Autodesk Fusion 360 part; units mm, degrees
(part 6 of 6)
  spline S266 degree 5 poles (46.3256, -26.1313) (46.3173, -26.12) (46.3005, -26.0976) (46.2753, -26.0639) (46.2416, -26.0191) (46.1993, -25.9633) (46.1569, -25.9077) (46.1143, -25.8522) (46.0715, -25.797) (46.0286, -25.7419) (45.9856, -25.687) (45.9424, -25.6324) (45.899, -25.5779) (45.8555, -25.5236) (45.8119, -25.4695) (45.768, -25.4156) (45.7241, -25.3619) (45.6799, -25.3084) (45.6356, -25.2552) (45.5912, -25.2021) (45.5466, -25.1492) (45.5018, -25.0966) (45.4569, -25.0441) (45.4118, -24.9919) (45.3665, -24.9399) (45.3211, -24.8881) (45.2755, -24.8365) (45.2297, -24.7851) (45.1838, -24.734) (45.1377, -24.6831) (45.0914, -24.6324) (45.045, -24.582) (44.9984, -24.5318) (44.9516, -24.4818) (44.9046, -24.4321) (44.8575, -24.3827) (44.8102, -24.3334) (44.7627, -24.2845) (44.7151, -24.2357) (44.6672, -24.1873) (44.6192, -24.1391) (44.571, -24.0912) (44.5226, -24.0435) (44.481, -24.003) (44.4491, -23.9721) (44.4268, -23.9507) (44.4144, -23.9388) (44.4117, -23.9362) knots -1 -1 -1 -1 -1 -1 -0.985714 -0.971429 -0.957143 -0.942857 -0.928571 -0.914286 -0.9 -0.885714 -0.871429 -0.857143 -0.842857 -0.828571 -0.814286 -0.8 -0.785714 -0.771429 -0.757143 -0.742857 -0.728571 -0.714286 -0.7 -0.685714 -0.671429 -0.657143 -0.642857 -0.628571 -0.614286 -0.6 -0.585714 -0.571429 -0.557143 -0.542857 -0.528571 -0.514286 -0.5 -0.485714 -0.471429 -0.457143 -0.442857 -0.428571 -0.414286 -0.4 -0.396066 -0.396066 -0.396066 -0.396066 -0.396066 -0.396066
  spline S267 degree 3 poles (44.3152, -23.3421) (44.2848, -23.3997) (44.266, -23.4627) (44.2536, -23.5923) (44.2602, -23.6577) (44.2914, -23.761) (44.309, -23.8002) (44.3538, -23.8731) (44.3808, -23.9066) (44.4117, -23.9362) knots 0 0 0 0 0.019532 0.019532 0.039064 0.039064 0.051902 0.051902 0.06474 0.06474 0.06474 0.06474
  arc A134 (44.3152, -23.3421) -> (44.5389, -22.9124) centre (0, 0) ccw
  spline S268 degree 3 poles (45.0809, -22.6507) (45.017, -22.638) (44.9513, -22.6379) (44.8235, -22.663) (44.7626, -22.6878) (44.6726, -22.7472) (44.64, -22.7753) (44.5828, -22.839) (44.5585, -22.8743) (44.5389, -22.9124) knots 0 0 0 0 0.019532 0.019532 0.039064 0.039064 0.051902 0.051902 0.06474 0.06474 0.06474 0.06474
  spline S269 degree 5 poles (45.0809, -22.6507) (45.0845, -22.6514) (45.1015, -22.6548) (45.1317, -22.6607) (45.1754, -22.6692) (45.2324, -22.68) (45.2992, -22.6923) (45.3661, -22.7043) (45.4331, -22.716) (45.5003, -22.7274) (45.5675, -22.7385) (45.6349, -22.7493) (45.7023, -22.7598) (45.7699, -22.77) (45.8375, -22.78) (45.9053, -22.7897) (45.9731, -22.799) (46.0411, -22.8081) (46.1091, -22.817) (46.1773, -22.8255) (46.2455, -22.8338) (46.3138, -22.8419) (46.3822, -22.8496) (46.4507, -22.8571) (46.5193, -22.8644) (46.5879, -22.8714) (46.6566, -22.8781) (46.7255, -22.8846) (46.7944, -22.8908) (46.8633, -22.8968) (46.9324, -22.9025) (47.0015, -22.908) (47.0707, -22.9132) (47.14, -22.9182) (47.2094, -22.9229) (47.2788, -22.9274) (47.3483, -22.9317) (47.4179, -22.9357) (47.4875, -22.9395) (47.5572, -22.9431) (47.627, -22.9464) (47.6968, -22.9495) (47.7667, -22.9523) (47.8367, -22.9549) (47.8927, -22.9569) (47.9347, -22.9582) (47.9628, -22.959) (47.9768, -22.9595) knots 0.396066 0.396066 0.396066 0.396066 0.396066 0.396066 0.4 0.414286 0.428571 0.442857 0.457143 0.471429 0.485714 0.5 0.514286 0.528571 0.542857 0.557143 0.571429 0.585714 0.6 0.614286 0.628571 0.642857 0.657143 0.671429 0.685714 0.7 0.714286 0.728571 0.742857 0.757143 0.771429 0.785714 0.8 0.814286 0.828571 0.842857 0.857143 0.871429 0.885714 0.9 0.914286 0.928571 0.942857 0.957143 0.971429 0.985714 1 1 1 1 1 1
  arc A135 (47.9768, -22.9595) -> (48.4269, -21.9943) centre (0, 0) ccw
  spline S270 degree 5 poles (48.4269, -21.9943) (48.4175, -21.9838) (48.3989, -21.9629) (48.3708, -21.9315) (48.3333, -21.8899) (48.2863, -21.8379) (48.2392, -21.7862) (48.192, -21.7347) (48.1446, -21.6834) (48.097, -21.6323) (48.0494, -21.5814) (48.0016, -21.5307) (47.9536, -21.4802) (47.9056, -21.4299) (47.8574, -21.3798) (47.809, -21.33) (47.7605, -21.2803) (47.7119, -21.2309) (47.6631, -21.1817) (47.6142, -21.1327) (47.5651, -21.0839) (47.5159, -21.0353) (47.4666, -20.987) (47.4171, -20.9389) (47.3675, -20.891) (47.3177, -20.8434) (47.2678, -20.796) (47.2178, -20.7488) (47.1676, -20.7019) (47.1172, -20.6552) (47.0667, -20.6087) (47.016, -20.5625) (46.9652, -20.5166) (46.9143, -20.4709) (46.8632, -20.4255) (46.8119, -20.3803) (46.7605, -20.3354) (46.7089, -20.2907) (46.6572, -20.2463) (46.6053, -20.2022) (46.5533, -20.1584) (46.501, -20.1149) (46.4487, -20.0716) (46.4038, -20.0349) (46.3692, -20.0069) (46.3452, -19.9875) (46.3318, -19.9767) (46.3288, -19.9744) knots -1 -1 -1 -1 -1 -1 -0.985714 -0.971429 -0.957143 -0.942857 -0.928571 -0.914286 -0.9 -0.885714 -0.871429 -0.857143 -0.842857 -0.828571 -0.814286 -0.8 -0.785714 -0.771429 -0.757143 -0.742857 -0.728571 -0.714286 -0.7 -0.685714 -0.671429 -0.657143 -0.642857 -0.628571 -0.614286 -0.6 -0.585714 -0.571429 -0.557143 -0.542857 -0.528571 -0.514286 -0.5 -0.485714 -0.471429 -0.457143 -0.442857 -0.428571 -0.414286 -0.4 -0.396066 -0.396066 -0.396066 -0.396066 -0.396066 -0.396066
  spline S271 degree 3 poles (46.1809, -19.391) (46.1557, -19.451) (46.1425, -19.5154) (46.1414, -19.6456) (46.1536, -19.7102) (46.1938, -19.8103) (46.2147, -19.8478) (46.2657, -19.9166) (46.2955, -19.9476) (46.3288, -19.9744) knots 0 0 0 0 0.019532 0.019532 0.039064 0.039064 0.051902 0.051902 0.06474 0.06474 0.06474 0.06474
  arc A136 (46.1809, -19.391) -> (46.3663, -18.9434) centre (0, 0) ccw
  spline S272 degree 3 poles (46.8834, -18.6354) (46.8187, -18.6284) (46.7532, -18.634) (46.6281, -18.6701) (46.5697, -18.7002) (46.4851, -18.7672) (46.4551, -18.798) (46.4037, -18.8664) (46.3825, -18.9038) (46.3663, -18.9434) knots 0 0 0 0 0.019532 0.019532 0.039064 0.039064 0.051902 0.051902 0.06474 0.06474 0.06474 0.06474
  spline S273 degree 5 poles (46.8834, -18.6354) (46.8872, -18.6358) (46.9043, -18.6377) (46.935, -18.641) (46.9792, -18.6456) (47.0369, -18.6514) (47.1046, -18.6578) (47.1723, -18.664) (47.2401, -18.6698) (47.3079, -18.6753) (47.3759, -18.6805) (47.4439, -18.6854) (47.5121, -18.69) (47.5802, -18.6943) (47.6485, -18.6983) (47.7169, -18.702) (47.7853, -18.7055) (47.8537, -18.7086) (47.9223, -18.7115) (47.9909, -18.7141) (48.0596, -18.7164) (48.1284, -18.7184) (48.1972, -18.7202) (48.2661, -18.7217) (48.335, -18.723) (48.404, -18.7239) (48.4731, -18.7246) (48.5422, -18.7251) (48.6114, -18.7253) (48.6806, -18.7252) (48.7499, -18.7249) (48.8192, -18.7243) (48.8886, -18.7235) (48.9581, -18.7224) (49.0276, -18.7211) (49.0971, -18.7196) (49.1667, -18.7177) (49.2364, -18.7157) (49.3061, -18.7134) (49.3758, -18.7109) (49.4456, -18.7081) (49.5155, -18.7051) (49.5854, -18.7018) (49.6553, -18.6984) (49.7113, -18.6954) (49.7533, -18.6931) (49.7813, -18.6914) (49.7953, -18.6906) knots 0.396066 0.396066 0.396066 0.396066 0.396066 0.396066 0.4 0.414286 0.428571 0.442857 0.457143 0.471429 0.485714 0.5 0.514286 0.528571 0.542857 0.557143 0.571429 0.585714 0.6 0.614286 0.628571 0.642857 0.657143 0.671429 0.685714 0.7 0.714286 0.728571 0.742857 0.757143 0.771429 0.785714 0.8 0.814286 0.828571 0.842857 0.857143 0.871429 0.885714 0.9 0.914286 0.928571 0.942857 0.957143 0.971429 0.985714 1 1 1 1 1 1
  arc A137 (49.7953, -18.6906) -> (50.1595, -17.6899) centre (0, 0) ccw
  spline S274 degree 5 poles (50.1595, -17.6899) (50.1493, -17.6803) (50.1289, -17.6611) (50.0982, -17.6323) (50.0572, -17.594) (50.0059, -17.5464) (49.9544, -17.499) (49.9029, -17.4518) (49.8512, -17.4048) (49.7994, -17.358) (49.7475, -17.3115) (49.6954, -17.2651) (49.6433, -17.219) (49.591, -17.1731) (49.5386, -17.1274) (49.4861, -17.082) (49.4335, -17.0367) (49.3807, -16.9917) (49.3278, -16.9469) (49.2748, -16.9024) (49.2217, -16.8581) (49.1685, -16.814) (49.1151, -16.7701) (49.0616, -16.7265) (49.008, -16.6832) (48.9543, -16.64) (48.9004, -16.5972) (48.8465, -16.5545) (48.7924, -16.5122) (48.7381, -16.47) (48.6838, -16.4282) (48.6293, -16.3866) (48.5747, -16.3452) (48.5199, -16.3041) (48.465, -16.2633) (48.41, -16.2228) (48.3549, -16.1825) (48.2996, -16.1426) (48.2442, -16.1029) (48.1887, -16.0634) (48.133, -16.0243) (48.0772, -15.9855) (48.0213, -15.947) (47.9733, -15.9143) (47.9365, -15.8894) (47.9109, -15.8722) (47.8965, -15.8626) (47.8934, -15.8605) knots -1 -1 -1 -1 -1 -1 -0.985714 -0.971429 -0.957143 -0.942857 -0.928571 -0.914286 -0.9 -0.885714 -0.871429 -0.857143 -0.842857 -0.828571 -0.814286 -0.8 -0.785714 -0.771429 -0.757143 -0.742857 -0.728571 -0.714286 -0.7 -0.685714 -0.671429 -0.657143 -0.642857 -0.628571 -0.614286 -0.6 -0.585714 -0.571429 -0.557143 -0.542857 -0.528571 -0.514286 -0.5 -0.485714 -0.471429 -0.457143 -0.442857 -0.428571 -0.414286 -0.4 -0.396066 -0.396066 -0.396066 -0.396066 -0.396066 -0.396066
  spline S275 degree 3 poles (47.6952, -15.2922) (47.6754, -15.3542) (47.6678, -15.4195) (47.6781, -15.5493) (47.6959, -15.6126) (47.7446, -15.7089) (47.7687, -15.7444) (47.8255, -15.8085) (47.8579, -15.8367) (47.8934, -15.8605) knots 0 0 0 0 0.019532 0.019532 0.039064 0.039064 0.051902 0.051902 0.06474 0.06474 0.06474 0.06474
  arc A138 (47.6952, -15.2922) -> (47.8409, -14.8302) centre (0, 0) ccw
  spline S276 degree 3 poles (48.3292, -14.4784) (48.2641, -14.477) (48.1994, -14.4883) (48.0779, -14.5351) (48.0223, -14.5702) (47.9439, -14.6443) (47.9167, -14.6776) (47.8715, -14.7502) (47.8536, -14.7893) (47.8409, -14.8302) knots 0 0 0 0 0.019532 0.019532 0.039064 0.039064 0.051902 0.051902 0.06474 0.06474 0.06474 0.06474
  spline S277 degree 5 poles (48.3292, -14.4784) (48.333, -14.4784) (48.3502, -14.4788) (48.3811, -14.4794) (48.4255, -14.4801) (48.4835, -14.4809) (48.5515, -14.4814) (48.6194, -14.4816) (48.6875, -14.4815) (48.7556, -14.4811) (48.8237, -14.4803) (48.8919, -14.4793) (48.9602, -14.4779) (49.0285, -14.4763) (49.0969, -14.4743) (49.1653, -14.4721) (49.2337, -14.4695) (49.3022, -14.4667) (49.3708, -14.4636) (49.4393, -14.4602) (49.508, -14.4565) (49.5766, -14.4525) (49.6453, -14.4483) (49.7141, -14.4438) (49.7829, -14.439) (49.8517, -14.434) (49.9206, -14.4287) (49.9895, -14.4231) (50.0584, -14.4173) (50.1274, -14.4112) (50.1964, -14.4048) (50.2654, -14.3982) (50.3345, -14.3913) (50.4035, -14.3842) (50.4727, -14.3768) (50.5418, -14.3692) (50.611, -14.3614) (50.6802, -14.3532) (50.7494, -14.3449) (50.8187, -14.3363) (50.888, -14.3274) (50.9573, -14.3183) (51.0266, -14.309) (51.096, -14.2995) (51.1515, -14.2916) (51.1931, -14.2856) (51.2209, -14.2816) (51.2348, -14.2796) knots 0.396066 0.396066 0.396066 0.396066 0.396066 0.396066 0.4 0.414286 0.428571 0.442857 0.457143 0.471429 0.485714 0.5 0.514286 0.528571 0.542857 0.557143 0.571429 0.585714 0.6 0.614286 0.628571 0.642857 0.657143 0.671429 0.685714 0.7 0.714286 0.728571 0.742857 0.757143 0.771429 0.785714 0.8 0.814286 0.828571 0.842857 0.857143 0.871429 0.885714 0.9 0.914286 0.928571 0.942857 0.957143 0.971429 0.985714 1 1 1 1 1 1
  arc A139 (51.2348, -14.2796) -> (51.5104, -13.2509) centre (0, 0) ccw
  spline S278 degree 5 poles (51.5104, -13.2509) (51.4994, -13.2422) (51.4774, -13.2248) (51.4443, -13.1988) (51.4002, -13.1643) (51.3449, -13.1213) (51.2895, -13.0786) (51.234, -13.0361) (51.1784, -12.9938) (51.1228, -12.9517) (51.067, -12.9098) (51.0111, -12.8682) (50.9551, -12.8268) (50.899, -12.7856) (50.8429, -12.7447) (50.7866, -12.704) (50.7302, -12.6635) (50.6737, -12.6232) (50.6172, -12.5832) (50.5605, -12.5435) (50.5037, -12.504) (50.4468, -12.4647) (50.3898, -12.4257) (50.3328, -12.3869) (50.2756, -12.3483) (50.2183, -12.3101) (50.1609, -12.272) (50.1034, -12.2343) (50.0458, -12.1968) (49.9881, -12.1596) (49.9303, -12.1226) (49.8724, -12.0859) (49.8144, -12.0495) (49.7563, -12.0133) (49.6981, -11.9774) (49.6397, -11.9419) (49.5813, -11.9065) (49.5228, -11.8715) (49.4641, -11.8368) (49.4053, -11.8024) (49.3465, -11.7683) (49.2875, -11.7345) (49.2284, -11.701) (49.1778, -11.6726) (49.139, -11.651) (49.1119, -11.6361) (49.0968, -11.6278) (49.0935, -11.626) knots -1 -1 -1 -1 -1 -1 -0.985714 -0.971429 -0.957143 -0.942857 -0.928571 -0.914286 -0.9 -0.885714 -0.871429 -0.857143 -0.842857 -0.828571 -0.814286 -0.8 -0.785714 -0.771429 -0.757143 -0.742857 -0.728571 -0.714286 -0.7 -0.685714 -0.671429 -0.657143 -0.642857 -0.628571 -0.614286 -0.6 -0.585714 -0.571429 -0.557143 -0.542857 -0.528571 -0.514286 -0.5 -0.485714 -0.471429 -0.457143 -0.442857 -0.428571 -0.414286 -0.4 -0.396066 -0.396066 -0.396066 -0.396066 -0.396066 -0.396066
  spline S279 degree 3 poles (48.8466, -11.0771) (48.8322, -11.1406) (48.8303, -11.2063) (48.8519, -11.3347) (48.8751, -11.3962) (48.932, -11.4879) (48.9592, -11.5212) (49.0213, -11.5801) (49.056, -11.6054) (49.0935, -11.626) knots 0 0 0 0 0.019532 0.019532 0.039064 0.039064 0.051902 0.051902 0.06474 0.06474 0.06474 0.06474
  arc A140 (48.8466, -11.0771) -> (48.9514, -10.6042) centre (0, 0) ccw
  spline S280 degree 3 poles (49.4072, -10.2111) (49.3422, -10.2154) (49.2787, -10.2323) (49.1618, -10.2896) (49.1094, -10.3293) (49.0378, -10.41) (49.0136, -10.4455) (48.9749, -10.5218) (48.9605, -10.5623) (48.9514, -10.6042) knots 0 0 0 0 0.019532 0.019532 0.039064 0.039064 0.051902 0.051902 0.06474 0.06474 0.06474 0.06474
  spline S281 degree 5 poles (49.4072, -10.2111) (49.4109, -10.2109) (49.4282, -10.2097) (49.4589, -10.2076) (49.5033, -10.2045) (49.5611, -10.2002) (49.6288, -10.1948) (49.6966, -10.189) (49.7644, -10.183) (49.8322, -10.1766) (49.9, -10.17) (49.9678, -10.163) (50.0357, -10.1557) (50.1036, -10.1481) (50.1715, -10.1402) (50.2395, -10.132) (50.3075, -10.1235) (50.3755, -10.1147) (50.4435, -10.1056) (50.5115, -10.0962) (50.5795, -10.0866) (50.6476, -10.0767) (50.7157, -10.0665) (50.7838, -10.056) (50.8519, -10.0452) (50.92, -10.0342) (50.9881, -10.0229) (51.0563, -10.0114) (51.1245, -9.9995) (51.1926, -9.9874) (51.2608, -9.9751) (51.329, -9.9625) (51.3972, -9.9496) (51.4654, -9.9365) (51.5336, -9.9232) (51.6019, -9.9095) (51.6701, -9.8957) (51.7383, -9.8816) (51.8066, -9.8672) (51.8748, -9.8526) (51.9431, -9.8377) (52.0113, -9.8226) (52.0796, -9.8073) (52.1478, -9.7917) (52.2025, -9.7791) (52.2434, -9.7695) (52.2707, -9.7631) (52.2844, -9.7598) knots 0.396066 0.396066 0.396066 0.396066 0.396066 0.396066 0.4 0.414286 0.428571 0.442857 0.457143 0.471429 0.485714 0.5 0.514286 0.528571 0.542857 0.557143 0.571429 0.585714 0.6 0.614286 0.628571 0.642857 0.657143 0.671429 0.685714 0.7 0.714286 0.728571 0.742857 0.757143 0.771429 0.785714 0.8 0.814286 0.828571 0.842857 0.857143 0.871429 0.885714 0.9 0.914286 0.928571 0.942857 0.957143 0.971429 0.985714 1 1 1 1 1 1
  arc A141 (52.2844, -9.7598) -> (52.4693, -8.7111) centre (0, 0) ccw
  spline S282 degree 5 poles (52.4693, -8.7111) (52.4576, -8.7034) (52.4341, -8.688) (52.3989, -8.665) (52.3519, -8.6344) (52.2931, -8.5964) (52.2342, -8.5587) (52.1752, -8.5211) (52.1162, -8.4838) (52.057, -8.4468) (51.9978, -8.4099) (51.9385, -8.3733) (51.8791, -8.337) (51.8197, -8.3008) (51.7602, -8.2649) (51.7006, -8.2293) (51.6409, -8.1939) (51.5811, -8.1587) (51.5212, -8.1238) (51.4613, -8.0891) (51.4013, -8.0547) (51.3412, -8.0205) (51.2811, -7.9866) (51.2208, -7.9529) (51.1605, -7.9196) (51.1001, -7.8864) (51.0396, -7.8535) (50.979, -7.8209) (50.9184, -7.7886) (50.8577, -7.7565) (50.7969, -7.7247) (50.736, -7.6932) (50.675, -7.662) (50.614, -7.6311) (50.5528, -7.6004) (50.4916, -7.57) (50.4303, -7.5399) (50.369, -7.5102) (50.3075, -7.4807) (50.246, -7.4515) (50.1844, -7.4227) (50.1227, -7.3941) (50.0609, -7.3659) (50.008, -7.342) (49.9674, -7.3239) (49.9392, -7.3114) (49.9234, -7.3045) (49.92, -7.303) knots -1 -1 -1 -1 -1 -1 -0.985714 -0.971429 -0.957143 -0.942857 -0.928571 -0.914286 -0.9 -0.885714 -0.871429 -0.857143 -0.842857 -0.828571 -0.814286 -0.8 -0.785714 -0.771429 -0.757143 -0.742857 -0.728571 -0.714286 -0.7 -0.685714 -0.671429 -0.657143 -0.642857 -0.628571 -0.614286 -0.6 -0.585714 -0.571429 -0.557143 -0.542857 -0.528571 -0.514286 -0.5 -0.485714 -0.471429 -0.457143 -0.442857 -0.428571 -0.414286 -0.4 -0.396066 -0.396066 -0.396066 -0.396066 -0.396066 -0.396066
  spline S283 degree 3 poles (49.6261, -6.7777) (49.6173, -6.8422) (49.6212, -6.9078) (49.6539, -7.0339) (49.6824, -7.0931) (49.7471, -7.1795) (49.777, -7.2103) (49.844, -7.2635) (49.8808, -7.2857) (49.92, -7.303) knots 0 0 0 0 0.019532 0.019532 0.039064 0.039064 0.051902 0.051902 0.06474 0.06474 0.06474 0.06474
  arc A142 (49.6261, -6.7777) -> (49.6893, -6.2974) centre (0, 0) ccw
  spline S284 degree 3 poles (50.1091, -5.8661) (50.0448, -5.876) (49.983, -5.8984) (49.8715, -5.9657) (49.8228, -6.0099) (49.7585, -6.0965) (49.7375, -6.134) (49.7055, -6.2134) (49.6947, -6.255) (49.6893, -6.2974) knots 0 0 0 0 0.019532 0.019532 0.039064 0.039064 0.051902 0.051902 0.06474 0.06474 0.06474 0.06474
  spline S285 degree 5 poles (50.1091, -5.8661) (50.1128, -5.8656) (50.1299, -5.8629) (50.1604, -5.8581) (50.2043, -5.8512) (50.2615, -5.8418) (50.3285, -5.8305) (50.3955, -5.8189) (50.4625, -5.807) (50.5295, -5.7947) (50.5965, -5.7822) (50.6635, -5.7693) (50.7304, -5.7561) (50.7974, -5.7426) (50.8644, -5.7288) (50.9314, -5.7147) (50.9984, -5.7003) (51.0653, -5.6857) (51.1323, -5.6707) (51.1992, -5.6554) (51.2662, -5.6399) (51.3331, -5.6241) (51.4, -5.608) (51.467, -5.5916) (51.5339, -5.575) (51.6008, -5.558) (51.6677, -5.5409) (51.7346, -5.5234) (51.8014, -5.5057) (51.8683, -5.4877) (51.9351, -5.4695) (52.002, -5.451) (52.0688, -5.4322) (52.1356, -5.4132) (52.2024, -5.3939) (52.2692, -5.3744) (52.3359, -5.3547) (52.4027, -5.3347) (52.4694, -5.3144) (52.5361, -5.2939) (52.6028, -5.2732) (52.6695, -5.2522) (52.7362, -5.231) (52.8028, -5.2095) (52.8561, -5.1921) (52.8961, -5.179) (52.9227, -5.1702) (52.936, -5.1658) knots 0.396066 0.396066 0.396066 0.396066 0.396066 0.396066 0.4 0.414286 0.428571 0.442857 0.457143 0.471429 0.485714 0.5 0.514286 0.528571 0.542857 0.557143 0.571429 0.585714 0.6 0.614286 0.628571 0.642857 0.657143 0.671429 0.685714 0.7 0.714286 0.728571 0.742857 0.757143 0.771429 0.785714 0.8 0.814286 0.828571 0.842857 0.857143 0.871429 0.885714 0.9 0.914286 0.928571 0.942857 0.957143 0.971429 0.985714 1 1 1 1 1 1
  arc A143 (52.936, -5.1658) -> (53.0289, -4.1049) centre (0, 0) ccw
  spline S286 degree 5 poles (53.0289, -4.1049) (53.0165, -4.0983) (52.9918, -4.085) (52.9547, -4.0651) (52.9052, -4.0388) (52.8433, -4.0061) (52.7814, -3.9736) (52.7193, -3.9413) (52.6573, -3.9093) (52.5951, -3.8776) (52.5329, -3.846) (52.4707, -3.8147) (52.4083, -3.7837) (52.346, -3.7529) (52.2835, -3.7223) (52.221, -3.692) (52.1585, -3.6619) (52.0959, -3.6321) (52.0332, -3.6025) (51.9705, -3.5732) (51.9077, -3.5441) (51.8449, -3.5153) (51.782, -3.4868) (51.719, -3.4585) (51.656, -3.4305) (51.593, -3.4027) (51.5299, -3.3753) (51.4667, -3.3481) (51.4035, -3.3211) (51.3402, -3.2945) (51.2768, -3.2681) (51.2134, -3.242) (51.15, -3.2162) (51.0865, -3.1907) (51.0229, -3.1655) (50.9593, -3.1406) (50.8956, -3.116) (50.8319, -3.0916) (50.7681, -3.0676) (50.7042, -3.0439) (50.6403, -3.0206) (50.5764, -2.9975) (50.5124, -2.9748) (50.4576, -2.9556) (50.4156, -2.9411) (50.3864, -2.9311) (50.37, -2.9256) (50.3665, -2.9244) knots -1 -1 -1 -1 -1 -1 -0.985714 -0.971429 -0.957143 -0.942857 -0.928571 -0.914286 -0.9 -0.885714 -0.871429 -0.857143 -0.842857 -0.828571 -0.814286 -0.8 -0.785714 -0.771429 -0.757143 -0.742857 -0.728571 -0.714286 -0.7 -0.685714 -0.671429 -0.657143 -0.642857 -0.628571 -0.614286 -0.6 -0.585714 -0.571429 -0.557143 -0.542857 -0.528571 -0.514286 -0.5 -0.485714 -0.471429 -0.457143 -0.442857 -0.428571 -0.414286 -0.4 -0.396066 -0.396066 -0.396066 -0.396066 -0.396066 -0.396066
  spline S287 degree 3 poles (50.028, -2.4267) (50.0248, -2.4918) (50.0344, -2.5568) (50.078, -2.6795) (50.1115, -2.736) (50.1835, -2.8164) (50.216, -2.8445) (50.2874, -2.8917) (50.326, -2.9106) (50.3665, -2.9244) knots 0 0 0 0 0.019532 0.019532 0.039064 0.039064 0.051902 0.051902 0.06474 0.06474 0.06474 0.06474
  line L0 (-1.6, 0) -> (-1.6, 2.0494)
  line L1 (-1.6, 0) -> (-1.6, -2.0494)
  line L2 (1.6, 0) -> (1.6, 2.0494)
  line L3 (1.6, 0) -> (1.6, -2.0494)
  arc A144 (-1.6, -2.0494) -> (1.6, -2.0494) centre (0, 0) ccw
  arc A145 (1.6, 2.0494) -> (-1.6, 2.0494) centre (0, 0) ccw
  constraint coincident A0.centre A1.centre
  constraint concentric A144 A145
extrude "Extrude3" cut sketch "Sketch4" along normal mid plane 16 contours L0 L1 L2 L3 A144 A145
named bodies: "Spur Gear (72 teeth)"
